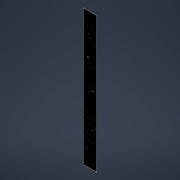
# Autodesk Inventor part: DarkSkyPanel
Saved by Autodesk Inventor 2021 (Build 250183000, 183)
## iProperties
Created: 2021-01-31
Part Number: DarkSkyPanel
Material: Generic
Document SubType Name: Modeling
Designer: argon
Density: 1 g/cm^3
Appearance: Anodized - Black
Author: argon
Autodesk Inventor part; units mm, degrees
ref_plane "YZ Plane" through (0, 0, 0) normal (1, 0, 0) x (0, 1, 0)
ref_plane "XZ Plane" through (0, 0, 0) normal (0, 1, 0) x (-1, 0, 0)
ref_plane "XY Plane" through (0, 0, 0) normal (0, 0, 1) x (1, 0, 0)
sketch "Sketch1" plane through (0, 0, 0) normal (0, 0, 1) x (1, 0, 0)
  line L0 (-695.173, 7000) -> (695.173, 7000)
  line L1 (695.173, 7000) -> (695.173, -7000)
  line L2 (695.173, -7000) -> (-695.173, -7000)
  line L3 (-695.173, -7000) -> (-695.173, 7000)
  line L4 (-695.173, 7000) -> (695.173, -7000) construction
  line L5 (695.173, 7000) -> (-695.173, -7000) construction
  point P0 (0, 0)
  dimension "d0" = 1390.346
  dimension "d1" = 14000
  constraints: 12 end point, 2 midpoint, 2 parallel, 1 horizontal, 1 perpendicular
  measures "d0" distance of L1.end L2.end
  measures "d1" distance of L0.end L1.end
extrude "Extrusion1" add sketch "Sketch1" along normal blind 1
sketch "Sketch2" plane through (0, 0, 1) normal (0, 0, 1) x (1, 0, 0)
  circle A0 centre (304.0961, 2079.1366) radius 11.1438
  circle A1 centre (-213.0977, 2833.9886) radius 48.1033
  circle A2 centre (189.8138, 3098.9022) radius 2.895
  circle A3 centre (124.7576, 3143.7051) radius 8.2342
  circle A4 centre (-184.4035, 4909.2967) radius 22.8684
  circle A5 centre (-609.6848, 4971.7787) radius 3.4163
  circle A6 centre (-295.8203, 5702.7273) radius 2.6539
  circle A7 centre (292.9522, 5730.0249) radius 8.308
  circle A8 centre (124.7576, 5373.9698) radius 2.3737
  circle A9 centre (525.5846, 4246.998) radius 14.7931
  circle A10 centre (-453.1844, 4393.0111) radius 8.6407
  circle A11 centre (-261.2009, 4474.8426) radius 8.0227
  circle A12 centre (-93.7676, 4627.2739) radius 3.5879
  circle A13 centre (32.991, 4652.9465) radius 10.148
  circle A14 centre (-133.1009, 227.9777) radius 8.8619
  circle A15 centre (-26.4949, 186.6367) radius 7.3446
  circle A16 centre (107.3406, 103.3976) radius 1.6321
  circle A17 centre (160.3852, 37.2959) radius 10.6403
  circle A18 centre (228.119, 0) radius 10.6089
  circle A19 centre (292.9522, 10.6089) radius 8.308
  circle A20 centre (370.1152, 57.6976) radius 12.7234
  circle A21 centre (265.6582, 441.2506) radius 14.2521
  circle A22 centre (-190.525, 426.9986) radius 6.1497
  circle A23 centre (-133.1009, -1024.8503) radius 6
  circle A24 centre (579.1583, -3225.3414) radius 12.4997
  circle A25 centre (265.6582, -3181.893) radius 6.2069
  circle A26 centre (-207.2719, -3101.2032) radius 10.3448
  circle A27 centre (-19.1502, -2867.4097) radius 2.069
  circle A28 centre (189.8138, -3014.3065) radius 8.2759
  circle A29 centre (160.3852, -2575.6851) radius 7.2414
  circle A30 centre (-217.6167, -2536.3747) radius 18.6494
  circle A31 centre (-483.2573, -2083.2705) radius 8.3403
  circle A32 centre (-236.2662, -5439.1351) radius 9.9685
  circle A33 centre (-293.1664, -5239.2916) radius 9.3483
  circle A34 centre (-599.6905, -5384.3016) radius 8.9652
  circle A35 centre (-330.7628, -5641.3649) radius 8.4411
  circle A36 centre (160.3852, -5551.7223) radius 10.2473
  circle A37 centre (315.2399, -4634.268) radius 10.4947
  circle A38 centre (124.7576, -4420.4023) radius 4.4555
  circle A39 centre (-93.7676, -4146.8325) radius 8.02
  circle A40 centre (-293.1664, -3853.6583) radius 10.3558
  circle A41 centre (315.2399, -3778.8053) radius 10.3558
  circle A42 centre (217.5101, -3518.602) radius 10.952
  circle A43 centre (-113.9095, -4568.1959) radius 10.211
  circle A44 centre (-444.5437, -4544.5165) radius 4.3053
  circle A45 centre (-518.6112, -4383.0664) radius 14.6397
  point P0 (0, 0)
  dimension "d4" = 12
  constraints: 46 centre point
  measures "d4" diameter of A23
extrude "Extrusion2" cut sketch "Sketch2" against normal through all
body "Solid1"
